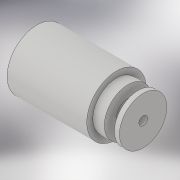
# Autodesk Inventor part: Deckel_klein
Saved by Autodesk Inventor 2018 (Build 220112000, 112)
## iProperties
Created: 2018-01-29
Part Number: Deckel_klein
Material: Generisch
Document SubType Name: Modeling
Designer: User
Density: 1 g/cm^3
Appearance: Vorgabe
Author: User
Autodesk Inventor part; units mm, degrees
ref_plane "YZ Plane" through (0, 0, 0) normal (1, 0, 0) x (0, 1, 0)
ref_plane "XZ Plane" through (0, 0, 0) normal (0, 1, 0) x (-1, 0, 0)
ref_plane "XY Plane" through (0, 0, 0) normal (0, 0, 1) x (1, 0, 0)
sketch "Skizze1" plane through (0, 0, 0) normal (0, 0, 1) x (1, 0, 0)
  line L0 (-10.54, 0) -> (63.24, 0) projected
  line L1 (0, -2.95) -> (0, 17.7) projected
  line L2 (0, 0) -> (0, 14.75)
  line L3 (0, 14.75) -> (39.5, 14.75)
  line L4 (39.5, 14.75) -> (39.5, 11.75)
  line L5 (39.5, 11.75) -> (45.2, 11.75)
  line L6 (45.2, 11.75) -> (45.2, 5.75)
  line L7 (45.2, 5.75) -> (50.2, 5.75)
  line L8 (50.2, 5.75) -> (50.2, 11.75)
  line L9 (50.2, 11.75) -> (52.7, 11.75)
  line L10 (52.7, 11.75) -> (52.7, 0)
  line L11 (0, 0) -> (52.7, 0)
  dimension "d0" = 14.75
  dimension "d2" = 3
  dimension "d4" = 6
  dimension "d5" = 5
  dimension "d6" = 2.5
  dimension "d12" = 5.7
  dimension "d13" = 39.5
  constraints: 20 end point, 8 perpendicular, 4 point on line
  measures "d0" distance of L2.start L2.end
  measures "d2" distance of L3.end L4.end
  measures "d4" distance of L5.end L6.end
  measures "d5" distance of L6.end L7.end
  measures "d6" distance of L8.end L9.end
  measures "d12" distance between parallel lines of L6 L4
  measures "d13" distance of L2.end L3.end
revolve "Umdrehung1" add sketch "Skizze1" angle 360 about axis through (-10, 0, 0) along (1, 0, 0)
sketch "Skizze2" plane through (52.7, 0, 0) normal (1, 0, 0) x (0, 0, -1)
  circle A0 centre (0, 0) radius 2.1
  dimension "d8" = 4.2
  constraints: 1 centre point, 1 coincident
  measures "d8" diameter of A0
extrude "Extrusion1" cut sketch "Skizze2" against normal blind 100
